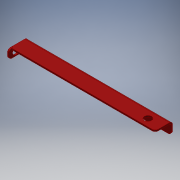
# Autodesk Inventor part: Lamiera pistone scarico
Saved by Autodesk Inventor 2018 (Build 220112000, 112)
## iProperties
Created: 2020-06-13
Part Number: Lamiera pistone scarico
Material: Generico
Document SubType Name: Lamiera
Designer: Francesco
Density: 1 g/cm^3
Sheet Metal Rule: Default_mm
Appearance: Rosso
Author: Francesco
Autodesk Inventor part; units mm, degrees
ref_plane "YZ Plane" through (0, 0, 0) normal (1, 0, 0) x (0, 1, 0)
ref_plane "XZ Plane" through (0, 0, 0) normal (0, 1, 0) x (-1, 0, 0)
ref_plane "XY Plane" through (0, 0, 0) normal (0, 0, 1) x (1, 0, 0)
sketch "Schizzo9" plane through (0, 0, 0) normal (0, 0, 1) x (1, 0, 0)
  line L0 (-50, 5) -> (50, 5)
  line L1 (50, 5) -> (50, -5)
  line L2 (50, -5) -> (-50, -5)
  line L3 (-50, -5) -> (-50, 5)
  line L4 (-50, 5) -> (50, -5) construction
  line L5 (50, 5) -> (-50, -5) construction
  point P0 (0, 0)
  dimension "d87" = 100
  dimension "d88" = 10
  measures "d87" distance of L1.end L2.end
  measures "d88" distance of L0.end L1.end
extrude "Piano6" add sketch "Schizzo9" along normal blind 1
sketch "Schizzo19" plane through (-50, 6, -1) normal (0, 1, 0) x (-1, 0, 0)
  line L0 (-100, 0) -> (0, 0)
  line L1 (0, 0) -> (0, 6)
  line L2 (0, 6) -> (-100, 6)
  line L3 (-100, 6) -> (-100, 0)
  constraints: 6 end point, 1 horizontal, 1 perpendicular, 1 vertical
edge flange "Flangia9" height 8 angle -90 thickness 1 bend radius 1 thickness toward (0, 1, 0) relief tear relief width 1 relief depth 0.5 edges at (0, 5, 1) wall of the first edge with corners at (50, 6, -1) (-50, 6, -1) (-50, 6, -7) (50, 6, -7)
bend "Piega (Bend)9"
corner "Angolo9"
sketch "Schizzo20" plane through (-51, 5, -1) normal (-1, 0, 0) x (0, 1, 0)
  line L0 (0, -6) -> (0, 0)
  line L1 (0, 0) -> (-10, 0)
  line L2 (-10, 0) -> (-10, -6)
  line L3 (-10, -6) -> (0, -6)
  constraints: 8 end point
edge flange "Flangia10" height 12 angle -90 thickness 1 bend radius 1 thickness toward (-1, 0, 0) relief tear relief width 1 relief depth 0.5 edges at (-50, 7, -4) wall of the first edge with corners at (-51, 5, -7) (-51, 5, -1) (-51, -5, -1) (-51, -5, -7)
bend "Piega (Bend)10"
corner "Angolo10"
sketch "Schizzo21" plane through (0, 0, 1) normal (0, 0, 1) x (1, 0, 0)
  line L0 (50, 5) -> (50, -5) projected
  point P0 (0, 0)
  point P1 (40, 0)
  point P2 (50, 0)
  dimension "d202" = 10
  constraints: 1 horizontal alignment, 1 midpoint
  measures "d202" distance of point (50, 0) point (40, 0)
hole "Foro7" at (40, 0, 1) direction (0, 0, -1) diameter 5 end through all
fillet "Arrotondamento angolo7" radius 2 5 edges at (50, 6.5, -7) (50, -5, 0.5) (-50, -5, 0.5) (-51.5, -5, -1) (-51.5, -5, -7)
sketch "Schizzo23" plane through (-52, 5, -7) normal (-1, 0, 0) x (0, 0, 1)
  line L0 (2, -10) -> (4, -10) projected
  point P0 (7, -5)
  point P1 (3, -5)
  point P2 (3, -10)
  constraints: 1 horizontal alignment, 1 midpoint, 1 vertical alignment
hole "Foro9" at (-52, 0, -4) direction (1, 0, 0) diameter 5 end through all
equation "\"d208\" = Spessore"
equation "\"d224\" = Spessore"
equation "\"d89\" = Spessore"
equation "\"d182\" = LarghezzaScaricoPiega"
equation "\"d183\" = ProfonditàScaricoPiega"
equation "\"d184\" = ResiduoMinimo"
equation "\"d185\" = RaggioTransizione"
equation "\"d188\" = RaggioPiega"
equation "\"d189\" = DimensioniScaricoAngolo"
equation "\"d190\" = DimensioneGioco"
equation "\"d191\" = Dimensione_raggio_Jacobi"
equation "\"d192\" = LarghezzaScaricoPiega"
equation "\"d193\" = ProfonditàScaricoPiega"
equation "\"d194\" = ResiduoMinimo"
equation "\"d195\" = RaggioTransizione"
equation "\"d198\" = RaggioPiega"
equation "\"d199\" = DimensioniScaricoAngolo"
equation "\"d200\" = DimensioneGioco"
equation "\"d201\" = Dimensione_raggio_Jacobi"
equation "\"RaggioPiega\" = Spessore"
equation "\"LarghezzaScaricoPiega\" = Spessore"
equation "\"ProfonditàScaricoPiega\" = 0.5 * Spessore"
equation "\"DimensioniScaricoAngolo\" = 4 * Spessore"
equation "\"ResiduoMinimo\" = 2 * Spessore"
equation "\"RaggioTransizione\" = RaggioPiega"
equation "\"Dimensione_raggio_Jacobi\" = RaggioPiega"
equation "\"DimensioneGioco\" = Spessore"
equation "\"Spessore\" = 1"
